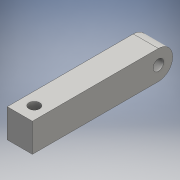
# Autodesk Inventor part: Puller
Saved by Autodesk Inventor 2016 (Build 200138000, 138)
## iProperties
Created: 2016-04-18
Part Number: Puller
Material: Generic
Document SubType Name: Modeling
Designer: amenoni
Density: 1 g/cm^3
Appearance: Default
Author: amenoni
Autodesk Inventor part; units mm, degrees
ref_plane "YZ Plane" through (0, 0, 0) normal (1, 0, 0) x (0, 1, 0)
ref_plane "XZ Plane" through (0, 0, 0) normal (0, 1, 0) x (-1, 0, 0)
ref_plane "XY Plane" through (0, 0, 0) normal (0, 0, 1) x (1, 0, 0)
sketch "Sketch1" plane through (0, 0, 0) normal (1, 0, 0) x (0, 1, 0)
  line L0 (-19.5584, -4) -> (19.5584, -4)
  line L1 (19.5584, -4) -> (19.5584, 4)
  line L2 (19.5584, 4) -> (-19.5584, 4)
  line L3 (-19.5584, 4) -> (-19.5584, -4)
  line L4 (-19.5584, -4) -> (19.5584, 4) construction
  line L5 (19.5584, -4) -> (-19.5584, 4) construction
  point P0 (0, 0)
  dimension "d0" = 8
  constraints: 12 end point, 2 midpoint, 2 parallel, 1 horizontal, 1 perpendicular
  measures "d0" distance of L1.end L0.end
extrude "Extrusion1" add sketch "Sketch1" along normal blind 7
sketch "Sketch2" plane through (7, 0, 0) normal (1, 0, 0) x (0, 0, -1)
  arc A0 (4, 15.5584) -> (-4, 15.5584) centre (0, 15.5584) ccw projected
  point P0 (0, 0)
  constraints: 1 coincident
fillet "Fillet2" radius 4 2 edges at (3.5, 19.5584, -4) (3.5, 19.5584, 4)
hole "Hole1" at (7, 15.5584, 0) direction (-1, 0, 0) diameter 3 end through all
sketch "Sketch3" plane through (0, -19.5584, 4) normal (0, 0, 1) x (1, 0, 0)
  line L0 (0, 0) -> (7, 0) projected
  point P0 (0, 19.5584)
  point P1 (3.5348, 4)
  dimension "d12" = 4
  measures "d12" distance from line of L0 point (3.535, 4)
hole "Hole2" at (3.5348, -15.5584, 4) direction (0, 0, -1) diameter 3 end through all
body "Solid1"
